Autodesk Fusion 360 part; units mm, degrees
(part 5 of 5)
equation "depthCuts = ceil(tempDepthPieces / 2)"
equation "shoulderToothDepth = ( depth - fingerWidth * tempDepthPieces ) / 2 - kerf"
equation "d48 = toolDiameter"
equation "d49 = boneCenterToHoleSide"
equation "d50 = shoulderToothDepth"
equation "d51 = thickness"
equation "d52 = boneCenterToHoleSide"
equation "d54 = boneCenterToHoleBottom"
equation "d55 = holeWidth"
equation "d56 = depthCuts"
equation "d58 = 2 * fingerWidth"
equation "d80 = depth"
equation "d82 = holeWidth"
equation "d85 = height"
equation "d86 = toolDiameter"
equation "d87 = boneCenterToHoleSide"
equation "d88 = boneCenterToHoleBottom"
equation "d89 = boneCenterToHoleSide"
equation "d98 = toolDiameter"
equation "d99 = shouderHoleDepth"
equation "d100 = thickness"
equation "tempHeightPieces = ceil(( ( floor(( height - 2 * thickness ) / fingerWidth) - 2 ) - ( ( floor(( height - 2 * thickness ) / fingerWidth) - 2 ) % 2 - 1 ) ))"
equation "heightCuts = ceil(tempHeightPieces / 2)"
equation "sholderToothHeight = ( height - fingerWidth * tempHeightPieces ) / 2 - kerf"
equation "d104 = thickness"
equation "d105 = holeWidth"
equation "d113 = toolDiameter"
equation "d114 = boneCenterToHoleBottom"
equation "d115 = boneCenterToHoleSide"
equation "d116 = toolDiameter"
equation "d117 = boneCenterToHoleSide"
equation "d119 = boneCenterToHoleSide"
equation "d122 = sholderToothHeight"
equation "d126 = thickness"
equation "d128 = heightCuts"
equation "d130 = -2 * fingerWidth"
equation "d132 = depthCuts - 2"
equation "d134 = -2 * fingerWidth"
equation "d140 = height"
equation "d141 = holeWidth"
equation "d142 = thickness"
equation "d143 = thickness"
equation "d144 = length"
equation "d145 = toolDiameter"
equation "d146 = boneCenterToHoleSide"
equation "d147 = boneCenterToHoleBottom"
equation "d148 = boneCenterToHoleSide"
equation "d149 = shoulderHoleHeight"
equation "d150 = thickness"
equation "d151 = thickness"
equation "d152 = holeWidth"
equation "d154 = toolDiameter"
equation "d155 = boneCenterToHoleBottom"
equation "d156 = boneCenterToHoleSide"
equation "d157 = toolDiameter"
equation "d159 = boneCenterToHoleSide"
equation "d160 = thickness"
equation "d163 = toolDiameter"
equation "d164 = boneCenterToHoleSide"
equation "d169 = thickness"
equation "d171 = fingerWidth - 2 * kerf"
equation "d172 = lengthCuts - 1"
equation "d174 = -2 * fingerWidth"
equation "d178 = heightCuts"
equation "d180 = -2 * fingerWidth"
equation "d182 = boneCenterToHoleSide"
equation "d183 = thickness"
equation "d184 = toolDiameter"
equation "d185 = toolDiameter"
equation "d186 = boneCenterToHoleSide"
equation "d187 = boneCenterToHoleSide"
equation "d189 = shoulderToothLength"
equation "d191 = shoulderHoleLength"
equation "d192 = fingerWidth - 2 * kerf"
equation "d193 = shoulderHoleLength"
equation "kerf = -0.095 mm"
equation "holeWidth = fingerWidth + 2 * kerf"
equation "shoulderHoleLength = shoulderToothLength + 2 * kerf"
equation "shouderHoleDepth = shoulderToothDepth + 2 * kerf"
equation "shoulderHoleHeight = sholderToothHeight + 2 * kerf"
equation "d354 = fingerWidth - 2 * kerf"
equation "assembleScrewDiam = 2.1 mm"
equation "assembleScrewDistance = 6 mm"
equation "assembleAvoidCollisionDistance = 1 mm"
equation "coolingHoleDistance = 8 mm"
equation "boneCornerToCenterPack = -3 * kerf"
equation "boneCenterToHoleSide = boneCenterToHoleBottom - boneCornerToCenterPack"
equation "d416 = boneCenterToHoleSide"
equation "d417 = shouderHoleDepth"
equation "d418 = shoulderHoleHeight"
equation "d442 = thickness"
equation "d473 = length"
equation "d474 = toolDiameter"
equation "d475 = depth"
equation "d476 = toolDiameter"
equation "d479 = -toolDiameter / 2"
equation "d282 = platformGrommetMountDiameter"
equation "d289 = pcbMountHoles"
equation "d422 = length"
equation "d423 = depth"
equation "d463 = toolDiameter + 0.1 mm"
equation "d843 = toolDiameter"
equation "d523 = depth"
equation "pumpLength = 52 mm"
equation "pumpCircleDiam = 30 mm"
equation "pumpHeight = 34 mm"
equation "sensorWireDistance = 10 mm"
equation "sensorWireDiam = 3.5 mm"
equation "pumpScrewDiam = 3 mm"
equation "d846 = hangerWireDiameter"
equation "d910 = depth"
equation "d911 = height"
equation "d930 = sensorWireDiam"
equation "d1194 = depth / 2"
equation "d993 = length + toolDiameter"
equation "d502 = length"
equation "d503 = height"
equation "d870 = ventDiameter"
equation "d1047 = toolDiameter"
equation "d1048 = 3 * toolDiameter"
equation "d492 = length"
equation "d493 = height"
equation "d1106 = toolDiameter"
equation "d1136 = depth"
equation "d1137 = height"
equation "d1162 = -topPillowHoleDistance"
equation "d1163 = length"
equation "d1164 = depth"
equation "d1173 = ventDiameter"
equation "d1177 = ( depth - topPillowHoleDistance ) / 2"
equation "d1086 = toolDiameter"
equation "d1087 = boneCenterToHoleSide"
equation "d1091 = fingerWidth - 2 * kerf"
equation "d1094 = toolDiameter"
equation "d1109 = boneCenterToHoleSide"
equation "d1113 = toolDiameter"
equation "d1116 = thickness"
equation "d1117 = boneCenterToHoleBottom"
equation "d1221 = toolDiameter"
equation "d1222 = toolDiameter"
equation "d1223 = toolDiameter"
equation "d1224 = toolDiameter"
equation "d1225 = toolDiameter"
equation "d1227 = boneCenterToHoleBottom"
equation "d1228 = boneCenterToHoleBottom"
equation "d1229 = boneCenterToHoleSide"
equation "d1230 = boneCenterToHoleSide"
equation "d1232 = boneCenterToHoleSide"
equation "d1233 = boneCenterToHoleSide"
equation "d1235 = boneCenterToHoleBottom"
equation "d1236 = boneCenterToHoleBottom"
equation "d1178 = boneCenterToHoleBottom"
equation "d1323 = length"
equation "d1376 = depthCuts"
equation "d1378 = 2 * fingerWidth"
equation "d1379 = toolDiameter"
equation "d1380 = boneCenterToHoleSide"
equation "d1381 = holeWidth"
equation "d1382 = toolDiameter"
equation "d1383 = shoulderToothDepth"
equation "d1384 = thickness"
equation "d1385 = toolDiameter"
equation "d1386 = toolDiameter"
equation "d1387 = boneCenterToHoleSide"
equation "d1388 = boneCenterToHoleSide"
equation "d1389 = boneCenterToHoleBottom"
equation "d1390 = boneCenterToHoleBottom"
equation "d1391 = boneCenterToHoleBottom"
equation "d1393 = boneCenterToHoleSide"
equation "d1395 = length"
equation "d1399 = toolDiameter"
equation "d1400 = toolDiameter"
equation "d1401 = length + toolDiameter"
equation "d1404 = toolDiameter"
equation "d1405 = boneCenterToHoleSide"
equation "d1406 = fingerWidth - 2 * kerf"
equation "d1407 = toolDiameter"
equation "d1408 = boneCenterToHoleSide"
equation "d1409 = toolDiameter"
equation "d1412 = boneCenterToHoleBottom"
equation "d1413 = toolDiameter"
equation "d1414 = toolDiameter"
equation "d1415 = toolDiameter"
equation "d1416 = toolDiameter"
equation "d1417 = toolDiameter"
equation "d1418 = boneCenterToHoleBottom"
equation "d1419 = boneCenterToHoleBottom"
equation "d1420 = boneCenterToHoleSide"
equation "d1421 = boneCenterToHoleSide"
equation "d1423 = boneCenterToHoleSide"
equation "d1424 = boneCenterToHoleSide"
equation "d1425 = boneCenterToHoleBottom"
equation "d1426 = boneCenterToHoleBottom"
equation "d1427 = boneCenterToHoleBottom"
equation "d1428 = length"
equation "d1431 = shoulderHoleHeight"
equation "d1433 = holeWidth"
equation "d1436 = toolDiameter"
equation "d1437 = shoulderHoleHeight"
equation "d1440 = 3 * toolDiameter"
equation "d1441 = boneCenterToHoleSide"
equation "d1442 = boneCenterToHoleSide"
equation "d1443 = boneCenterToHoleBottom"
equation "d1444 = boneCenterToHoleBottom"
equation "d1446 = thickness"
equation "d1447 = thickness"
equation "d1451 = thickness"
equation "d1452 = height"
equation "d1453 = thickness"
equation "d1454 = thickness"
equation "d1456 = boneCenterToHoleSide"
equation "d1457 = boneCenterToHoleSide"
equation "d1460 = height"
equation "d1461 = toolDiameter"
equation "d1462 = thickness"
equation "d1463 = thickness"
equation "d1466 = holeWidth"
equation "d1468 = shoulderHoleHeight"
equation "d1469 = shoulderHoleHeight"
equation "d1472 = boneCenterToHoleBottom"
equation "d1473 = boneCenterToHoleBottom"
equation "pcbMountHoles = 2 mm"
equation "d1481 = toolDiameter"
equation "d1482 = boneCenterToHoleSide"
equation "d1483 = holeWidth"
equation "d1484 = toolDiameter"
equation "d1485 = shoulderToothDepth"
equation "d1486 = thickness"
equation "d1487 = toolDiameter"
equation "d1488 = toolDiameter"
equation "d1489 = boneCenterToHoleSide"
equation "d1490 = boneCenterToHoleSide"
equation "d1491 = boneCenterToHoleBottom"
equation "d1492 = boneCenterToHoleBottom"
equation "d1493 = boneCenterToHoleBottom"
equation "d1495 = boneCenterToHoleSide"
equation "d1496 = depth"
equation "d1497 = length"
equation "d1515 = platformGrommetMountDiameter"
equation "d1516 = platformGrommetMountDiameter"
equation "d1517 = platformGrommetMountDiameter"
equation "d1518 = platformGrommetMountDiameter"
equation "ventDiameter = 3 mm"
equation "d1542 = height"
equation "platformGrommetMountDiameter = 3.5 mm"
equation "d1557 = platformGrommetMountDiameter"
equation "d1558 = platformGrommetMountDiameter"
equation "d1559 = platformGrommetMountDiameter"
equation "d1560 = platformGrommetMountDiameter"
equation "d1561 = sensorWireDiam"
equation "d1567 = 11 mm + thickness"
equation "d1571 = toolDiameter"
equation "d1573 = toolDiameter"
equation "d1574 = boneCenterToHoleBottom"
equation "d1575 = boneCenterToHoleBottom"
equation "d1576 = boneCenterToHoleSide"
equation "d1577 = boneCenterToHoleSide"
equation "d1578 = toolDiameter"
equation "d1579 = toolDiameter"
equation "d1580 = boneCenterToHoleSide"
equation "d1581 = boneCenterToHoleSide"
equation "d1582 = boneCenterToHoleBottom"
equation "d1583 = boneCenterToHoleBottom"
equation "d1584 = toolDiameter"
equation "d1585 = toolDiameter"
equation "d1586 = boneCenterToHoleBottom"
equation "d1587 = boneCenterToHoleSide"
equation "d1588 = boneCenterToHoleSide"
equation "d1589 = boneCenterToHoleBottom"
equation "d1590 = toolDiameter"
equation "d1591 = toolDiameter"
equation "d1592 = boneCenterToHoleBottom"
equation "d1593 = boneCenterToHoleBottom"
equation "d1594 = boneCenterToHoleSide"
equation "d1595 = boneCenterToHoleSide"
equation "d1609 = thickness"
equation "d1618 = thickness"
equation "d1621 = depth + toolDiameter"
equation "d1622 = depth"
equation "d1640 = 48 mm + thickness - ( 49 / 2 ) * 1 mm"
equation "hangerWireDiameter = 2 mm"
equation "topPillowHoleDistance = 22 mm"
equation "d1675 = pumpCircleDiam"
equation "d1677 = pumpHeight"
equation "d1678 = pumpLength"
equation "d1679 = ( pumpHeight - pumpScrewDiam ) / 2"
equation "d1680 = pumpScrewDiam"
equation "d1696 = ventDiameter"
equation "d1705 = ventDiameter"
equation "d1716 = thickness"
equation "d1722 = toolDiameter"
equation "d1726 = toolDiameter + 0.001 mm"
equation "d1748 = pumpScrewDiam"
equation "d1754 = ( 41 / 2 ) * 1 mm + thickness + 2 mm"
equation "d1757 = -41 mm - 6 mm"
equation "d1766 = pumpScrewDiam"
equation "d1783 = 360.0 °"
equation "d1796 = holeWidth"
equation "d1797 = thickness"
equation "d1798 = thickness"
equation "d1799 = toolDiameter"
equation "d1800 = boneCenterToHoleSide"
equation "d1801 = boneCenterToHoleBottom"
equation "d1802 = boneCenterToHoleSide"
equation "d1803 = toolDiameter"
equation "d1804 = boneCenterToHoleSide"
equation "d1805 = shoulderToothDepth"
equation "d1806 = thickness"
equation "d1807 = boneCenterToHoleSide"
equation "d1808 = boneCenterToHoleBottom"
equation "d1809 = holeWidth"
equation "d1810 = depth"
equation "d1811 = holeWidth"
equation "d1812 = height"
equation "d1813 = toolDiameter"
equation "d1814 = boneCenterToHoleSide"
equation "d1815 = boneCenterToHoleBottom"
equation "d1816 = boneCenterToHoleSide"
equation "d1817 = toolDiameter"
equation "d1818 = shouderHoleDepth"
equation "d1819 = thickness"
equation "d1820 = thickness"
equation "d1821 = holeWidth"
equation "d1822 = toolDiameter"
equation "d1823 = boneCenterToHoleBottom"
equation "d1824 = boneCenterToHoleSide"
equation "d1825 = toolDiameter"
equation "d1826 = boneCenterToHoleSide"
equation "d1827 = boneCenterToHoleSide"
equation "d1828 = sholderToothHeight"
equation "d1829 = height"
equation "d1830 = holeWidth"
equation "d1831 = thickness"
equation "d1832 = thickness"
equation "d1833 = length"
equation "d1834 = toolDiameter"
equation "d1835 = boneCenterToHoleSide"
equation "d1836 = boneCenterToHoleBottom"
equation "d1837 = boneCenterToHoleSide"
equation "d1838 = shoulderHoleHeight"
equation "d1839 = thickness"
equation "d1840 = thickness"
equation "d1841 = holeWidth"
equation "d1842 = toolDiameter"
equation "d1843 = boneCenterToHoleBottom"
equation "d1844 = boneCenterToHoleSide"
equation "d1845 = toolDiameter"
equation "d1846 = boneCenterToHoleSide"
equation "d1847 = thickness"
equation "d1848 = toolDiameter"
equation "d1849 = boneCenterToHoleSide"
equation "d1850 = fingerWidth - 2 * kerf"
equation "d1851 = boneCenterToHoleSide"
equation "d1852 = thickness"
equation "d1853 = toolDiameter"
equation "d1854 = toolDiameter"
equation "d1855 = boneCenterToHoleSide"
equation "d1856 = boneCenterToHoleSide"
equation "d1857 = shoulderToothLength"
equation "d1858 = shoulderHoleLength"
equation "d1859 = fingerWidth - 2 * kerf"
equation "d1860 = shoulderHoleLength"
equation "d1861 = fingerWidth - 2 * kerf"
equation "d1862 = boneCenterToHoleSide"
equation "d1863 = shouderHoleDepth"
equation "d1864 = shoulderHoleHeight"
equation "d1865 = thickness"
equation "d1866 = length"
equation "d1867 = toolDiameter"
equation "d1868 = depth"
equation "d1869 = toolDiameter"
equation "d1887 = toolDiameter"
equation "d1888 = boneCenterToHoleSide"
equation "d1889 = boneCenterToHoleBottom"
equation "d1890 = boneCenterToHoleSide"
equation "d1896 = toolDiameter"
equation "d1899 = toolDiameter"
equation "d1926 = thickness"
equation "d1948 = boneCenterToHoleBottom"
equation "d1949 = boneCenterToHoleSide"
equation "d1951 = boneCenterToHoleSide"
equation "d1953 = holeWidth"
equation "d1956 = fingerWidth - 2 * kerf"
equation "d1958 = boneCenterToHoleSide"
equation "d1959 = boneCenterToHoleBottom"
equation "d1960 = boneCenterToHoleBottom"
equation "d1961 = holeWidth"
equation "d1962 = fingerWidth - 2 * kerf"
equation "d1963 = length + toolDiameter"
equation "d1965 = thickness"
equation "d1974 = depth / 2"
equation "d1975 = shouderHoleDepth"
equation "d1976 = fingerWidth - 2 * kerf"
equation "d1979 = depth / 2"
equation "d1982 = thickness"
equation "d1984 = height / 2 + toolDiameter + length"
equation "d1989 = sholderToothHeight"
equation "d1991 = depthCuts - 1"
equation "d1992 = 2 * fingerWidth"
equation "d1993 = 2 * fingerWidth"
equation "d1995 = depthCuts - 1"
equation "d1997 = 2 * fingerWidth"
equation "d2002 = heightCuts"
equation "d2004 = 2 * fingerWidth"
equation "d2006 = heightCuts"
equation "d2008 = 2 * fingerWidth"
equation "d2012 = extraLine"
equation "extraLine = ( max(-( fingerWidth - 2 * kerf ) + ( sholderToothHeight - thickness ); 0.001 mm) )"
equation "tempTrailingLineUnused = fingerWidth - 2 * kerf"
named bodies: "Side", "Box Front", "Box Top", "Box Right", "Front (1)", "Box Right Side (1)", "Box Bottom (1)", "Box Bottom", "Box  Left", "Box Back", "Brace", "Platform", "Box Top (1)"
